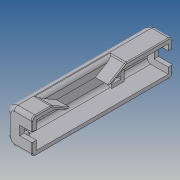
# Autodesk Inventor part: 5V_Supply
Saved by Autodesk Inventor 2019.4 (Build 234330000, 330)
## iProperties
Part Number: 5V_Supply
Material: GEDA Stahl
Document SubType Name: Modeling
Designer: Admin
Mass: 66.3821 g
Surface Area: 73.0202 cm^2
Volume: 8.44556 cm^3
Density: 7.86 g/cm^3
Appearance: GEDA Stahl A
Author: Admin
Gewicht: 0,066 kg
G_L: 0
G_H: 0
G_B: 0
InventorVersion: 2019.4
VAULT_Status: in Bearbeitung
Revision: -
Max. Breite: 0
Max. Höhe: 0
Max. Länge: 0
Max. Abmessungen: 0 x 0 x 0
Autodesk Inventor part; units mm, degrees
note: some values were not read from the file. Left out: dimensions or parameters whose unit could not be read.
ref_plane "YZ Plane" through (0, 0, 0) normal (1, 0, 0) x (0, 1, 0)
ref_plane "XZ Plane" through (0, 0, 0) normal (0, 1, 0) x (-1, 0, 0)
ref_plane "XY Plane" through (0, 0, 0) normal (0, 0, 1) x (1, 0, 0)
sketch "Skizze1" plane through (0, 0, 0) normal (1, 0, 0) x (0, 1, 0)
  line L0 (40, -10) -> (-40, -10)
  line L1 (-40, -10) -> (-40, 10)
  line L2 (-40, 10) -> (40, 10)
  line L3 (40, 10) -> (40, -10)
  line L4 (40, -10) -> (-40, 10) construction
  line L5 (-40, -10) -> (40, 10) construction
  point P0 (0, 0)
  dimension "d0" = 80
  dimension "d1" = 20
  constraints: 12 end point, 2 midpoint, 2 parallel, 1 horizontal, 1 perpendicular
  measures "d0" distance of L1.end L2.end
  measures "d1" distance of L0.end L1.end
extrude "Extrusion1" add sketch "Skizze1" along normal blind 14
sketch "Skizze2" plane through (14, 0, 0) normal (1, 0, 0) x (0, 0, -1)
  line L0 (7.5, 37.5) -> (-7.5, 37.5)
  line L1 (-7.5, 37.5) -> (-7.5, -37.5)
  line L2 (-7.5, -37.5) -> (7.5, -37.5)
  line L3 (7.5, -37.5) -> (7.5, 37.5)
  line L4 (7.5, 37.5) -> (-7.5, -37.5) construction
  line L5 (-7.5, 37.5) -> (7.5, -37.5) construction
  line L6 (10, 40) -> (-10, 40) projected
  point P0 (0, 0)
  dimension "d4" = 15
  dimension "d5" = 2.5
  constraints: 12 end point, 2 midpoint, 2 parallel, 1 horizontal, 1 perpendicular
  measures "d4" distance between parallel lines of L3 L1
  measures "d5" distance between parallel lines of L6 L0
extrude "Extrusion2" cut sketch "Skizze2" against normal blind 12
sketch "Skizze3" plane through (14, 0, 0) normal (1, 0, 0) x (0, 0, -1)
  line L0 (-2.7, -40) -> (2.5, -40)
  line L1 (2.5, -40) -> (2.5, -37.5)
  line L2 (2.5, -37.5) -> (-2.7, -37.5)
  line L3 (-2.7, -37.5) -> (-2.7, -40)
  line L4 (7.5, -37.5) -> (-7.5, -37.5) projected
  line L5 (-10, -40) -> (10, -40) projected
  line L6 (7.5, 37.5) -> (7.5, -37.5) projected
  point P0 (0, 0)
  dimension "d8" = 5.2
  dimension "d9" = 5
  constraints: 8 end point, 2 collinear, 2 parallel, 1 horizontal, 1 perpendicular
  measures "d8" distance between parallel lines of L1 L3
  measures "d9" distance between parallel lines of L6 L1
extrude "Extrusion3" cut sketch "Skizze3" against normal blind 7
sketch "Skizze4" plane through (2, 0, 0) normal (1, 0, 0) x (0, 0, -1)
  line L0 (5.5, -37.5) -> (7.5, -37.5)
  line L1 (7.5, -37.5) -> (7.5, -32.5)
  line L2 (7.5, -32.5) -> (5.5, -32.5)
  line L3 (5.5, -32.5) -> (5.5, -37.5)
  line L4 (7.5, -37.5) -> (-7.5, -37.5) projected
  line L5 (7.5, 37.5) -> (7.5, -37.5) projected
  line L6 (3.7, -37.5) -> (-7.5, -37.5)
  line L7 (-7.5, -37.5) -> (-7.5, -32.5)
  line L8 (-7.5, -32.5) -> (3.7, -32.5)
  line L9 (3.7, -32.5) -> (3.7, -37.5)
  line L10 (-7.5, -37.5) -> (-7.5, 37.5) projected
  line L11 (7.5, 14.5) -> (5.5, 14.5)
  line L12 (5.5, 14.5) -> (5.5, 19.5)
  line L13 (5.5, 19.5) -> (7.5, 19.5)
  line L14 (7.5, 19.5) -> (7.5, 14.5)
  line L15 (3.7, 14.5) -> (-7.5, 14.5)
  line L16 (-7.5, 14.5) -> (-7.5, 19.5)
  line L17 (-7.5, 19.5) -> (3.7, 19.5)
  line L18 (3.7, 19.5) -> (3.7, 14.5)
  line L19 (7.5, 19.5) -> (-7.5, 19.5)
  line L20 (-7.5, 19.5) -> (-7.5, 21.5)
  line L21 (-7.5, 21.5) -> (7.5, 21.5)
  line L22 (7.5, 21.5) -> (7.5, 19.5)
  point P0 (0, 0)
  dimension "d12" = 5
  dimension "d13" = 2
  dimension "d14" = 1.8
  dimension "d15" = 57
  dimension "d24" = 2
  constraints: 40 end point, 10 parallel, 7 collinear, 6 point on line, 5 horizontal, 5 perpendicular
  measures "d12" distance of L2.end L0.start
  measures "d13" distance between parallel lines of L1 L3
  measures "d14" distance between parallel lines of L9 L3
  measures "d15" distance between parallel lines of L17 L4
  measures "d24" distance of L19.end L20.end
extrude "Extrusion4" add sketch "Skizze4" along normal blind 3 contours L3 L2 L1 L0 | L4 L7 L8 L9 | L11 L12 L13 L5 | L13 L19 L17 L10 L21 L5 | L10 L17 L18 L15
fillet "Rundung1" radius 2 4 edges at (2, -9, 7.5) (2, -9, -7.5) (2, 29.5, 7.5) (2, 29.5, -7.5)
fillet "Rundung2" radius 4 2 edges at (0, 0, 10) (0, 0, -10)
sketch "Skizze5" plane through (14, 0, 0) normal (1, 0, 0) x (0, 0, -1)
  line L0 (-4, 37.5) -> (4, 37.5)
  line L1 (4, 37.5) -> (4, 40)
  line L2 (4, 40) -> (-4, 40)
  line L3 (-4, 40) -> (-4, 37.5)
  line L4 (-7.5, 37.5) -> (7.5, 37.5) projected
  line L5 (10, 40) -> (-10, 40) projected
  line L6 (-6, 40) -> (6, 40) projected
  point P0 (0, 0)
  point P1 (0, 40)
  point P2 (0, 40)
  dimension "d20" = 8
  constraints: 8 end point, 2 collinear, 2 midpoint, 2 parallel, 1 coincident, 1 horizontal, 1 perpendicular
  measures "d20" distance between parallel lines of L1 L3
extrude "Extrusion5" cut sketch "Skizze5" against normal blind 8
fillet "Rundung3" radius 2 10 edges at (0, 40, 0) (1.1716, 40, -8.8284) (9, 40, -10) (1.1716, 40, 8.8284) (9, 40, 10) (1.1716, -40, 8.8284) (9, -40, 10) (1.1716, -40, -8.8284) (9, -40, -10) (0, -40, 0)
sketch "Skizze6" plane through (14, 0, 0) normal (1, 0, 0) x (0, 0, -1)
  line L0 (-7.5, -37.5) -> (-7.5, 37.5) projected
  line L1 (-7.5, -26.7158) -> (-7.5, 11.7158)
  line L2 (-7.5, 11.7158) -> (-4.2, 6)
  line L3 (-7.5, -26.7158) -> (-4.2, -21)
  line L4 (-4.2, -21) -> (-4.2, 6)
  line L5 (-7.5, -7.5) -> (-4.2, -7.5) construction
  line L6 (-2.7, -40) -> (-2.7, -37.5) construction
  line L7 (-8, -40) -> (-2.7, -40) construction
  point P0 (0, 0)
  dimension "d25" = 27
  dimension "d26" = 30
  dimension "d27" = 1.5
  dimension "d28" = 19
  constraints: 10 end point, 2 midpoint, 2 point on line, 1 horizontal, 1 parallel, 1 other
  measures "d25" distance of L3.end L2.end
  measures "d26" angle of L4 L3
  measures "d27" distance between parallel lines of L6 L4
  measures "d28" distance from line of L3.end L7
extrude "Extrusion6" add sketch "Skizze6" against normal up to next
sketch "Skizze7" plane through (14, 0, 0) normal (1, 0, 0) x (0, 0, -1)
  line L0 (-4.2, 6) -> (-4.2, -21) projected
  line L1 (-4.2, -18.5) -> (-10, -28.5459)
  line L2 (-10, -38) -> (-10, 38) projected
  line L3 (-4.2, 3.5) -> (-10, 13.5459)
  line L4 (-10, 13.5459) -> (-10, -28.5459)
  line L5 (-4.2, 3.5) -> (-4.2, -18.5)
  line L6 (-10, -7.5) -> (-4.2, -7.5) construction
  line L7 (-4.2, -21) -> (-7.5, -26.7158) projected
  point P0 (0, 0)
  dimension "d31" = 22
  constraints: 10 end point, 3 midpoint, 2 parallel, 2 point on line, 1 coincident, 1 horizontal, 1 vertical, 1 other
  measures "d31" distance of L3.start L1.start
extrude "Extrusion7" cut sketch "Skizze7" against normal blind 7.5
fillet "Rundung4" radius 2 1 edges at (6.5, -7.5, 10)
fillet "Rundung6" radius 2 4 edges at (5.5, -28.5459, 10) (10.25, -28.5459, 10) (5.5, 13.5459, 10) (10.25, 13.5459, 10)
fillet "Rundung5" radius 0.5 11 edges at (14, -39.4142, 9.4142) (14, -40, 5.35) (14, -33.5409, 10) (14, 39.4142, 9.4142) (14, 40, 6) (14, 26.0409, 10) (14, 39.4142, -9.4142) (14, 40, -6) (14, -39.4142, -9.4142) (14, -40, -5.25) (14, 0, -10)
equation "\"G_L\" = 0"
equation "\"G_H\" = 0"
equation "\"G_B\" = 0"
